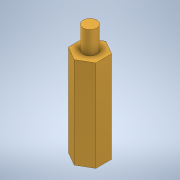
# Autodesk Inventor part: espaçador sext. 20mm
Saved by Autodesk Inventor 2021 (Build 250183000, 183)
## iProperties
Created: 2022-02-21
Part Number: espaçador sext. 20mm
Material: Generic
Document SubType Name: Modeling
Designer: Matheus
Density: 4.34112 g/cm^3
Appearance: Default
Mass: 2.4 g
Surface Area: 6.66542 cm^2
Volume: 0.552852 cm^3
Author: Matheus
Autodesk Inventor part; units mm, degrees
ref_plane "YZ Plane" through (0, 0, 0) normal (1, 0, 0) x (0, 1, 0)
ref_plane "XZ Plane" through (0, 0, 0) normal (0, 1, 0) x (-1, 0, 0)
ref_plane "XY Plane" through (0, 0, 0) normal (0, 0, 1) x (1, 0, 0)
sketch "Sketch1" plane through (0, 0, 0) normal (0, 1, 0) x (-1, 0, 0)
  circle A0 centre (0, 0) radius 1.5
  line L0 (-3, -1.7321) -> (-3, 1.7321)
  line L1 (-3, 1.7321) -> (0, 3.4641)
  line L2 (0, 3.4641) -> (3, 1.7321)
  line L3 (3, 1.7321) -> (3, -1.7321)
  line L4 (3, -1.7321) -> (0, -3.4641)
  line L5 (0, -3.4641) -> (-3, -1.7321)
  dimension "d0" = 3
  dimension "d1" = 6
  constraints: 12 end point, 2 coincident, 1 centre point, 1 vertical, 13 other
  measures "d0" diameter of A0
  measures "d1" distance between parallel lines of L3 L0
extrude "Extrusion1" add sketch "Sketch1" along normal blind 20
sketch "Sketch2" plane through (0, 20, 0) normal (0, 1, 0) x (1, 0, 0)
  circle A0 centre (0, 0) radius 1.5 construction
  circle A1 centre (0, 0) radius 1.5
  dimension "d4" = 3
  constraints: 1 centre point, 1 coincident
  measures "d4" diameter of A1
extrude "Extrusion2" add sketch "Sketch2" along normal mid plane 10
body "Solid1"
